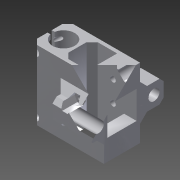
# Autodesk Inventor part: XEnd
Saved by Autodesk Inventor 2015 (Build 190159000, 159)
## iProperties
Created: 2014-08-10
Part Number: XEnd
Material: ABS Plastic
Document SubType Name: Modeling
Designer: Jack
Density: 1.06 g/cm^3
Appearance: Smooth - White
Author: Jack
Autodesk Inventor part; units mm, degrees
ref_plane "YZ Plane" through (0, 0, 0) normal (1, 0, 0) x (0, 1, 0)
ref_plane "XZ Plane" through (0, 0, 0) normal (0, 1, 0) x (-1, 0, 0)
ref_plane "XY Plane" through (0, 0, 0) normal (0, 0, 1) x (1, 0, 0)
sketch "Sketch1" plane through (0, 0, 0) normal (0, 0, 1) x (1, 0, 0)
  arc A0 (-7.8581, -1.5) -> (-7.8581, 1.5) centre (0, 0) ccw
  line L0 (-10, 13) -> (42, 13)
  line L1 (-7.8581, 1.5) -> (-10, 1.5)
  line L2 (-10, 1.5) -> (-10, 13)
  line L3 (-7.8581, -1.5) -> (-10, -1.5)
  line L4 (-10, -1.5) -> (-10, -13)
  line L5 (-10, -13) -> (42, -13)
  line L6 (42, 13) -> (42, -13)
  point P0 (0, 13)
  point P1 (-10, 9.0418)
  point P2 (0, -13)
  dimension "d0" = 16
  dimension "d5" = 1.5
  dimension "d7" = 13
  dimension "d12" = 10
  dimension "d13" = 1.5
  dimension "d14" = 13
  dimension "d15" = 52
  constraints: 14 end point, 5 vertical alignment, 4 horizontal, 3 point on line, 2 point on circle, 2 vertical, 1 centre point, 1 coincident, 1 perpendicular
  measures "d0" diameter of A0
  measures "d5" distance from line of point (0, 0) L1
  measures "d7" distance from line of point (0, 0) L0
  measures "d12" horizontal distance of A0.centre L1.end
  measures "d13" distance from line of point (0, 0) L3
  measures "d14" distance from line of point (0, 0) L5
  measures "d15" distance from line of L0.end L2
extrude "Extrusion1" add sketch "Sketch1" along normal blind 50
chamfer "Chamfer1" distance 4 angle 45 2 edges at (-10, 13, 25) (-10, -13, 25)
sketch "Sketch5" plane through (0, 0, 50) normal (0, 0, 1) x (1, 0, 0)
  line L0 (42, 13) -> (-6, 13) projected
  arc A0 (-7.8581, -1.5) -> (-7.8581, 1.5) centre (0, 0) ccw projected
  line L1 (10, -10.5) -> (28, -10.5)
  line L2 (28, -10.5) -> (28, 10.5)
  line L3 (28, 10.5) -> (10, 10.5)
  line L4 (10, 10.5) -> (10, -10.5)
  dimension "d36" = 18
  dimension "d37" = 21
  dimension "d38" = 10
  dimension "d39" = 2.5
  constraints: 8 end point, 2 parallel, 1 horizontal, 1 perpendicular
  measures "d36" distance of L2.end L3.end
  measures "d37" distance of L3.end L1.start
  measures "d38" distance from line of A0.centre L4
  measures "d39" distance between parallel lines of L0 L3
extrude "Extrusion5" cut sketch "Sketch5" against normal up to next
sketch "Sketch7" plane through (42, -13, 0) normal (1, 0, 0) x (0, 0, -1)
  line L0 (0, 0) -> (0, 26) projected
  line L1 (0, 26) -> (-50, 26) projected
  line L2 (-35, 2.5) -> (-15, 2.5)
  line L3 (-15, 2.5) -> (-15, 23.5)
  line L4 (-15, 23.5) -> (-35, 23.5)
  line L5 (-35, 23.5) -> (-35, 2.5)
  point P0 (0, 13)
  dimension "d49" = 20
  dimension "d50" = 21
  dimension "d51" = 2.5
  dimension "d52" = 15
  constraints: 8 end point, 2 parallel, 1 horizontal, 1 perpendicular
  measures "d49" distance of L3.end L4.end
  measures "d50" distance of L4.end L2.start
  measures "d51" distance between parallel lines of L1 L4
  measures "d52" distance between parallel lines of L0 L3
extrude "Extrusion7" cut sketch "Sketch7" against normal up to surface (14 mm away)
chamfer "Chamfer2" distance 5 angle 45 2 edges at (28, 0, 15) (28, 0, 35)
sketch "Sketch8" plane through (42, -13, 0) normal (1, 0, 0) x (0, 0, -1)
  line L0 (0, 26) -> (-50, 26) projected
  line L1 (0, 0) -> (-50, 0) projected
  circle A0 centre (-25, 36) radius 4
  circle A1 centre (-25, -4) radius 4
  line L2 (-33, 31) -> (-33, 43)
  line L3 (-33, 43) -> (-17, 43)
  line L4 (-17, 43) -> (-17, 31)
  line L5 (-33, -5) -> (-33, -11)
  line L6 (-33, -11) -> (-17, -11)
  line L7 (-17, -11) -> (-17, -5)
  line L8 (0, 0) -> (0, 26) projected
  line L9 (-38, 26) -> (-50, 26)
  line L10 (-12, 0) -> (0, 0)
  line L11 (-38, 0) -> (-50, 0)
  line L12 (-12, 26) -> (0, 26)
  line L13 (-38, 26) -> (-33, 31)
  line L14 (-17, 31) -> (-12, 26)
  line L15 (-17, -5) -> (-12, 0)
  line L16 (-38, 0) -> (-33, -5)
  line L17 (-38, 26) -> (-12, 26)
  line L18 (-38, 0) -> (-12, 0)
  point P0 (0, 13)
  point P1 (-33, 26)
  point P2 (-17, 26)
  point P3 (-33, 0)
  point P4 (-17, 0)
  dimension "d58" = 8
  dimension "d59" = 8
  dimension "d60" = 40
  dimension "d61" = 10
  dimension "d62" = 25
  dimension "d63" = 8
  dimension "d64" = 8
  dimension "d65" = 7
  dimension "d66" = 7
  dimension "d69" = 5
  dimension "d70" = 5
  dimension "d71" = 5
  dimension "d72" = 5
  dimension "d73" = 5
  dimension "d74" = 5
  dimension "d75" = 5
  dimension "d76" = 5
  constraints: 32 end point, 14 point on line, 5 perpendicular, 4 collinear, 2 centre point, 2 vertical alignment, 1 horizontal, 1 vertical
  measures "d58" diameter of A0
  measures "d59" diameter of A1
  measures "d60" distance of A1.centre A0.centre
  measures "d61" distance from line of L0 A0.centre
  measures "d62" horizontal distance of L0.start A0.centre
  measures "d63" distance from line of A1.centre L7
  measures "d64" distance from line of L5 A1.centre
  measures "d65" distance from line of A1.centre L6
  measures "d66" distance from line of A0.centre L3
  measures "d69" distance of L9.start point (-33, 26)
  measures "d70" distance of L2.start point (-33, 26)
  measures "d71" distance of L4.end point (-17, 26)
  measures "d72" distance of L12.start point (-17, 26)
  measures "d73" distance of L7.end point (-17, 0)
  measures "d74" distance of L10.start point (-17, 0)
  measures "d75" distance of L11.start point (-33, 0)
  measures "d76" distance of L5.start point (-33, 0)
extrude "Extrusion8" add sketch "Sketch8" against normal blind 26
chamfer "Chamfer3" distance 5 angle 45 3 edges at (16, 13, 25) (16, -13, 18.5) (16, -13, 31.5)
chamfer "Chamfer4" distance 3 angle 45 4 edges at (29, 30, 33) (29, 30, 17) (29, -24, 33) (29, -24, 17)
sketch "Sketch9" plane through (42, 30, 30) normal (0, 1, 0) x (1, 0, 0)
  line L0 (-31, 18) -> (0, 18) projected
  line L1 (0, 30) -> (0, 18) projected
  line L2 (0, 30) -> (-48, 30) projected
  line L3 (-48, -20) -> (-48, 30) projected
  line L4 (0, -20) -> (-48, -20) projected
  line L5 (0, -8) -> (0, -20) projected
  line L6 (0, -8) -> (-31, -8) projected
  line L7 (-31, 18) -> (-31, -8) projected
  line L8 (0, 18) -> (0, 13) projected
  line L9 (-31, 18) -> (0, 18) projected
  line L10 (-26, 13) -> (-31, 18) projected
  line L11 (0, 13) -> (-26, 13) projected
  line L12 (0, -3) -> (0, -8) projected
  line L13 (0, -3) -> (-26, -3) projected
  line L14 (-31, -8) -> (-26, -3) projected
  line L15 (0, -8) -> (-31, -8) projected
  circle A0 centre (-17, 12.5) radius 2
  circle A1 centre (-17, -2.5) radius 2
  line L16 (-52, 30) -> (-52, -20) projected
  point P0 (-42, 30)
  dimension "d83" = 4
  dimension "d84" = 4
  dimension "d85" = 15
  dimension "d86" = 35
  dimension "d97" = 17.5
  constraints: 2 centre point, 1 vertical alignment
  measures "d83" diameter of A0
  measures "d84" diameter of A1
  measures "d85" distance of A0.centre A1.centre
  measures "d86" distance from line of L16 A0.centre
  measures "d97" distance from line of L2 A0.centre
extrude "Extrusion9" cut sketch "Sketch9" against normal up to surface (54 mm away) contours A0 L11 | L11 A0 | A1 L13 | L13 A1
sketch "Sketch10" plane through (42, 30, 30) normal (0, 1, 0) x (1, 0, 0)
  circle A0 centre (-17, 12.5) radius 2 projected
  arc A1 (-18.9365, 13) -> (-15.0635, 13) centre (-17, 12.5) ccw projected
  arc A2 (-15.0635, 13) -> (-18.9365, 13) centre (-17, 12.5) ccw projected
  circle A3 centre (-17, -2.5) radius 2 projected
  arc A4 (-15.0635, -3) -> (-18.9365, -3) centre (-17, -2.5) ccw projected
  arc A5 (-18.9365, -3) -> (-15.0635, -3) centre (-17, -2.5) ccw projected
  circle A6 centre (-17, 12.5) radius 3.5
  circle A7 centre (-17, -2.5) radius 3.5
  point P0 (-42, 30)
  dimension "d89" = 7
  dimension "d90" = 7
  constraints: 2 centre point, 2 coincident
  measures "d89" diameter of A6
  measures "d90" diameter of A7
extrude "Extrusion10" cut sketch "Sketch10" against normal up to surface (17 mm away)
sketch "Sketch11" plane through (42, -24, 20) normal (0, -1, 0) x (1, 0, 0)
  arc A0 (-18.9365, 13) -> (-15.0635, 13) centre (-17, 12.5) ccw projected
  arc A1 (-15.0635, 13) -> (-18.9365, 13) centre (-17, 12.5) ccw projected
  circle A2 centre (-17, 12.5) radius 2 projected
  arc A3 (-15.0635, -3) -> (-18.9365, -3) centre (-17, -2.5) ccw projected
  arc A4 (-18.9365, -3) -> (-15.0635, -3) centre (-17, -2.5) ccw projected
  circle A5 centre (-17, -2.5) radius 2 projected
  line L0 (-12.9585, 12.5) -> (-14.9793, 9)
  line L1 (-14.9793, 9) -> (-19.0207, 9)
  line L2 (-19.0207, 9) -> (-21.0415, 12.5)
  line L3 (-21.0415, 12.5) -> (-19.0207, 16)
  line L4 (-19.0207, 16) -> (-14.9793, 16)
  line L5 (-14.9793, 16) -> (-12.9585, 12.5)
  line L6 (-12.9585, -2.5) -> (-14.9793, -6)
  line L7 (-14.9793, -6) -> (-19.0207, -6)
  line L8 (-19.0207, -6) -> (-21.0415, -2.5)
  line L9 (-21.0415, -2.5) -> (-19.0207, 1)
  line L10 (-19.0207, 1) -> (-14.9793, 1)
  line L11 (-14.9793, 1) -> (-12.9585, -2.5)
  point P0 (-42, -20)
  dimension "d93" = 7
  dimension "d94" = 7
  constraints: 24 end point, 2 coincident, 2 horizontal, 26 other
  measures "d93" distance between parallel lines of L7 L10
  measures "d94" distance between parallel lines of L4 L1
extrude "Extrusion11" cut sketch "Sketch11" against normal up to surface (11 mm away)
sketch "Sketch12" plane through (-6, 13, 0) normal (0, 1, 0) x (1, 0, 0)
  line L0 (48, 0) -> (0, 0) projected
  line L1 (48, -50) -> (0, -50) projected
  line L2 (-4, -50) -> (0, -50) projected
  line L3 (0, -50) -> (0, 0) projected
  line L4 (0, 0) -> (-4, 0) projected
  line L5 (-4, 0) -> (-4, -50) projected
  line L6 (-1.25, -1.7746) -> (1.5, -3.3623)
  line L7 (1.5, -3.3623) -> (1.5, -6.5377)
  line L8 (1.5, -6.5377) -> (-1.25, -8.1254)
  line L9 (-1.25, -8.1254) -> (-4, -6.5377)
  line L10 (-4, -6.5377) -> (-4, -3.3623)
  line L11 (-4, -3.3623) -> (-1.25, -1.7746)
  line L12 (-1.25, -41.8746) -> (1.5, -43.4623)
  line L13 (1.5, -43.4623) -> (1.5, -46.6377)
  line L14 (1.5, -46.6377) -> (-1.25, -48.2254)
  line L15 (-1.25, -48.2254) -> (-4, -46.6377)
  line L16 (-4, -46.6377) -> (-4, -43.4623)
  line L17 (-4, -43.4623) -> (-1.25, -41.8746)
  point P0 (6, 0)
  point P1 (-1.25, -4.95)
  point P2 (-1.25, -45.05)
  dimension "d98" = 5.5
  dimension "d99" = 5.5
  dimension "d100" = 0
  dimension "d101" = 0
  dimension "d102" = 4.95
  dimension "d103" = 4.95
  constraints: 24 end point, 2 vertical, 26 other
  measures "d98" distance between parallel lines of L13 L16
  measures "d99" distance between parallel lines of L7 L10
  measures "d100" distance between parallel lines of L5 L16
  measures "d101" distance between parallel lines of L5 L10
  measures "d102" distance from line of L0 point (-1.25, -4.95)
  measures "d103" distance from line of L1 point (-1.25, -45.05)
extrude "Extrusion12" cut sketch "Sketch12" against normal blind 4 contours L5 L17 L12 L3 L14 L15 | L3 L12 L13 L14 | L5 L11 L6 L3 L8 L9 | L3 L6 L7 L8
sketch "Sketch13" plane through (-6, 9, 0) normal (0, 1, 0) x (1, 0, 0)
  line L0 (-1.25, -41.8746) -> (1.5, -43.4623) projected
  line L1 (-4, -43.4623) -> (-1.25, -41.8746) projected
  line L2 (-1.25, -48.2254) -> (-4, -46.6377) projected
  line L3 (1.5, -46.6377) -> (-1.25, -48.2254) projected
  line L4 (1.5, -43.4623) -> (1.5, -46.6377) projected
  circle A0 centre (-1.25, -4.9498) radius 1.5
  circle A1 centre (-1.25, -45.0498) radius 1.5
  line L5 (-4, -43.4623) -> (-4, -46.6377) projected
  point P0 (1.5, -3.3623)
  point P1 (-1.25, -8.1254)
  point P2 (6, 0)
  dimension "d106" = 3
  dimension "d107" = 3
  dimension "d108" = 1.5875
  dimension "d109" = 1.5875
  constraints: 2 centre point, 2 vertical alignment
  measures "d106" diameter of A0
  measures "d107" diameter of A1
  measures "d108" vertical distance of point (1.5, -3.362) A0.centre
  measures "d109" vertical distance of L0.end A1.centre
extrude "Extrusion13" cut sketch "Sketch13" against normal blind 24.2 contours A0 | A1
sketch "Sketch14" plane through (-6, -13, 0) normal (0, -1, 0) x (1, 0, 0)
  arc A0 (0, 4.1206) -> (0, 5.7789) centre (-1.25, 4.9498) ccw projected
  arc A1 (0, 5.7789) -> (0, 4.1206) centre (-1.25, 4.9498) ccw projected
  arc A2 (-1.8581, 6.321) -> (-1.8581, 3.5786) centre (-1.25, 4.9498) ccw projected
  spline S0 degree 7 poles (-1.8581, 3.5786) (-1.8196, 3.5615) (-1.7751, 3.5433) (-1.7245, 3.5246) (-1.6678, 3.5064) (-1.6049, 3.4896) (-1.5358, 3.4753) (-1.3566, 3.4499) (-1.2409, 3.4422) (-1.1132, 3.4445) (-0.9735, 3.4609) (-0.8227, 3.4962) (-0.6632, 3.5567) (-0.4521, 3.6783) (-0.4025, 3.7098) (-0.3531, 3.7444) (-0.304, 3.7823) (-0.2555, 3.8237) (-0.2081, 3.8686) (-0.1359, 3.9447) (-0.1102, 3.9734) (-0.0851, 4.0032) (-0.0606, 4.0341) (-0.0368, 4.0662) (-0.0137, 4.0993) (0.0241, 4.1577) (0.0394, 4.1824) (0.0541, 4.2075) (0.0684, 4.2332) (0.0822, 4.2593) (0.0954, 4.286) (0.1889, 4.4853) (0.2469, 4.6756) (0.276, 4.8782) (0.2715, 5.0851) (0.2341, 5.2858) (0.1686, 5.4722) (0.0665, 5.6695) (0.0503, 5.6988) (0.0335, 5.7274) (0.0161, 5.7554) (-0.0018, 5.7827) (-0.0203, 5.8094) (-0.0672, 5.8734) (-0.0961, 5.91) (-0.1259, 5.9451) (-0.1565, 5.9785) (-0.1877, 6.0103) (-0.2194, 6.0406) (-0.3138, 6.1247) (-0.3775, 6.1743) (-0.4418, 6.2181) (-0.5063, 6.2566) (-0.5705, 6.2901) (-0.6338, 6.319) (-0.8201, 6.393) (-0.9399, 6.4257) (-1.0534, 6.4451) (-1.1598, 6.4539) (-1.2588, 6.4545) (-1.3503, 6.4488) (-1.5154, 6.4284) (-1.5894, 6.414) (-1.6566, 6.3967) (-1.717, 6.3777) (-1.7707, 6.3581) (-1.8177, 6.3389) (-1.8581, 6.321) knots 0 0 0 0 0 0 0 0 0.134403 0.134403 0.134403 0.134403 0.134403 0.134403 0.320085 0.320085 0.320085 0.320085 0.320085 0.320085 0.376676 0.376676 0.376676 0.376676 0.376676 0.376676 0.408759 0.408759 0.408759 0.408759 0.408759 0.408759 0.431365 0.431365 0.431365 0.431365 0.431365 0.431365 0.57527 0.57527 0.57527 0.57527 0.57527 0.57527 0.601005 0.601005 0.601005 0.601005 0.601005 0.601005 0.638924 0.638924 0.638924 0.638924 0.638924 0.638924 0.71242 0.71242 0.71242 0.71242 0.71242 0.71242 0.859157 0.859157 0.859157 0.859157 0.859157 0.859157 1 1 1 1 1 1 1 1 projected
  arc A3 (0, 44.2206) -> (0, 45.8789) centre (-1.25, 45.0498) ccw projected
  arc A4 (0, 45.8789) -> (0, 44.2206) centre (-1.25, 45.0498) ccw projected
  arc A5 (-1.8581, 46.421) -> (-1.8581, 43.6786) centre (-1.25, 45.0498) ccw projected
  spline S1 degree 7 poles (-1.8581, 43.6786) (-1.8196, 43.6615) (-1.7751, 43.6433) (-1.7245, 43.6246) (-1.6678, 43.6064) (-1.6049, 43.5896) (-1.5358, 43.5753) (-1.3566, 43.5499) (-1.2409, 43.5422) (-1.1132, 43.5445) (-0.9735, 43.5609) (-0.8227, 43.5962) (-0.6632, 43.6567) (-0.4521, 43.7783) (-0.4025, 43.8098) (-0.3531, 43.8444) (-0.304, 43.8823) (-0.2555, 43.9237) (-0.2081, 43.9686) (-0.1359, 44.0447) (-0.1102, 44.0734) (-0.0851, 44.1032) (-0.0606, 44.1341) (-0.0368, 44.1662) (-0.0137, 44.1993) (0.0241, 44.2577) (0.0394, 44.2824) (0.0541, 44.3075) (0.0684, 44.3332) (0.0822, 44.3593) (0.0954, 44.386) (0.1889, 44.5853) (0.2469, 44.7756) (0.276, 44.9782) (0.2715, 45.1851) (0.2341, 45.3858) (0.1686, 45.5722) (0.0665, 45.7695) (0.0503, 45.7988) (0.0335, 45.8274) (0.0161, 45.8554) (-0.0018, 45.8827) (-0.0203, 45.9094) (-0.0672, 45.9734) (-0.0961, 46.01) (-0.1259, 46.0451) (-0.1565, 46.0785) (-0.1877, 46.1103) (-0.2194, 46.1406) (-0.3138, 46.2247) (-0.3775, 46.2743) (-0.4418, 46.3181) (-0.5063, 46.3566) (-0.5705, 46.3901) (-0.6338, 46.419) (-0.8201, 46.493) (-0.9399, 46.5257) (-1.0534, 46.5451) (-1.1598, 46.5539) (-1.2588, 46.5545) (-1.3503, 46.5488) (-1.5154, 46.5284) (-1.5894, 46.514) (-1.6566, 46.4967) (-1.717, 46.4777) (-1.7707, 46.4581) (-1.8177, 46.4389) (-1.8581, 46.421) knots 0 0 0 0 0 0 0 0 0.134403 0.134403 0.134403 0.134403 0.134403 0.134403 0.320085 0.320085 0.320085 0.320085 0.320085 0.320085 0.376676 0.376676 0.376676 0.376676 0.376676 0.376676 0.408758 0.408758 0.408758 0.408758 0.408758 0.408758 0.431365 0.431365 0.431365 0.431365 0.431365 0.431365 0.57527 0.57527 0.57527 0.57527 0.57527 0.57527 0.601005 0.601005 0.601005 0.601005 0.601005 0.601005 0.638924 0.638924 0.638924 0.638924 0.638924 0.638924 0.71242 0.71242 0.71242 0.71242 0.71242 0.71242 0.859157 0.859157 0.859157 0.859157 0.859157 0.859157 1 1 1 1 1 1 1 1 projected
  circle A6 centre (-1.25, 4.9498) radius 2.75
  circle A7 centre (-1.25, 45.0498) radius 2.75
  point P0 (6, 0)
  dimension "d112" = 5.5
  dimension "d113" = 5.5
  constraints: 2 centre point, 2 coincident, 2 vertical alignment
  measures "d112" diameter of A6
  measures "d113" diameter of A7
extrude "Extrusion14" cut sketch "Sketch14" against normal blind 4
chamfer "Chamfer5" distance 4 angle 45 2 edges at (10, -10.5, 25) (10, 10.5, 25)
equation "\"d70\" = d69"
equation "\"d71\" = d69"
equation "\"d72\" = d71"
equation "\"d73\" = d69"
equation "\"d74\" = d73"
equation "\"d75\" = d69"
equation "\"d76\" = d75"
body "Solid1"
